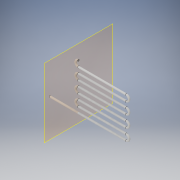
# Autodesk Inventor part: serpInf
Saved by Autodesk Inventor 2019.4 (Build 234330000, 330)
## iProperties
Created: 2020-04-11
Part Number: serpInf
Material: Genérico
Document SubType Name: Modeling
Designer: lucas
Density: 1 g/cm^3
Appearance: Padrão
Author: lucas
Autodesk Inventor part; units mm, degrees
ref_plane "XZ Plane" through (0, 0, 0) normal (0, 1, 0) x (-1, 0, 0)
ref_plane "XY Plane" through (0, 0, 0) normal (0, 0, 1) x (1, 0, 0)
sketch "Esboço3" plane through (0, 0, 0) normal (0, 0, 1) x (1, 0, 0)
  line L0 (0, 0) -> (1000, 0)
  line L1 (1000, 0) -> (1000, 1000)
  line L2 (1000, 1000) -> (0, 1000)
  line L3 (0, 1000) -> (0, 0)
  line L4 (80, 50) -> (920, 50)
  arc A0 (920, 50) -> (920, 150) centre (920, 100) ccw
  line L5 (920, 150) -> (80, 150)
  arc A1 (80, 250) -> (80, 150) centre (80, 200) ccw
  line L6 (80, 250) -> (920, 250)
  arc A2 (920, 250) -> (920, 350) centre (920, 300) ccw
  line L7 (920, 350) -> (80, 350)
  arc A3 (80, 450) -> (80, 350) centre (80, 400) ccw
  line L8 (80, 450) -> (920, 450)
  arc A4 (920, 450) -> (920, 550) centre (920, 500) ccw
  line L9 (920, 550) -> (80, 550)
  arc A5 (80, 650) -> (80, 550) centre (80, 600) ccw
  line L10 (80, 650) -> (920, 650)
  arc A6 (920, 650) -> (920, 750) centre (920, 700) ccw
  line L11 (920, 750) -> (80, 750)
  arc A7 (80, 850) -> (80, 750) centre (80, 800) ccw
  line L12 (80, 850) -> (1072.3642, 850)
  dimension "d18" = 1000
  dimension "d19" = 1000
  dimension "d20" = 50
  dimension "d21" = 50
  dimension "d23" = 50
  dimension "d24" = 80
  dimension "d25" = 80
  dimension "d28" = 200
  dimension "d33" = 80
  constraints: 26 end point, 16 point on circle, 8 centre point, 3 horizontal, 3 parallel, 3 tangent, 1 perpendicular, 1 vertical, 33 other
  measures "d18" distance of L1.end L2.end
  measures "d19" distance of L2.end L0.start
  measures "d20" radius of A1
  measures "d21" radius of A0
  measures "d23" distance between parallel lines of L0 L4
  measures "d24" distance from line of L1 A0.centre
  measures "d25" distance from line of A1.centre L3
  measures "d28" distance of L4.start L6.start
  measures "d33" distance from line of L3 L4.start
ref_plane "Plano de trabalho3" through (80, 50, 0) normal (1, 0, 0) x (0, 1, 0)
sketch "Esboço5" plane through (80, 50, 0) normal (1, 0, 0) x (0, 1, 0)
  circle A0 centre (0, 0) radius 15.525
  circle A1 centre (0, 0) radius 9.525
  point P0 (-50, 0)
  dimension "d36" = 19.05
  dimension "d37" = 6
  constraints: 2 centre point, 2 coincident
  measures "d36" diameter of A1
  measures "d37" radial gap between concentric circles of A0 A1
sweep "Varredura1" add profiles "Esboço5" path "Esboço3" path curves L4 A0 L5 A1
pattern_linear "Padrão retangular1" count 4 spacing 200 along (0, 1, 0) of "Varredura1"
sketch "Esboço6" plane through (80, 50, 0) normal (-1, 0, 0) x (0, 0, 1)
  circle A0 centre (0, 0) radius 9.525 projected
  circle A1 centre (0, 0) radius 15.525 projected
  point P0 (0, -50)
extrude "Extrusão1" add sketch "Esboço6" along normal blind 500
